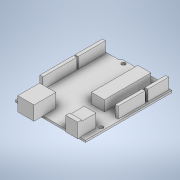
# Autodesk Inventor part: Arduino UNO
Saved by Autodesk Inventor 2020 (Build 240168000, 168)
## iProperties
Created: 2021-04-04
Part Number: Arduino UNO
Material: Типовые
Document SubType Name: Modeling
Designer: Антон
Density: 1 g/cm^3
Appearance: По умолчанию
Author: Антон
Autodesk Inventor part; units mm, degrees
ref_plane "YZ Plane" through (0, 0, 0) normal (1, 0, 0) x (0, 1, 0)
ref_plane "XZ Plane" through (0, 0, 0) normal (0, 1, 0) x (-1, 0, 0)
ref_plane "XY Plane" through (0, 0, 0) normal (0, 0, 1) x (1, 0, 0)
sketch "Эскиз1" plane through (0, 0, 0) normal (0, 1, 0) x (-1, 0, 0)
  line L0 (0, 0) -> (53.5, 0)
  line L1 (53.5, 0) -> (53.5, -66)
  line L2 (53.5, -66) -> (0, -66)
  line L3 (0, -66) -> (0, 0)
  line L4 (53.5, -66) -> (40.5, -66)
  line L5 (40.5, -66) -> (3, -66)
  line L6 (3, -66) -> (3, -67.5)
  line L7 (3, -67.5) -> (40.5, -67.5)
  line L8 (40.5, -67.5) -> (40.5, -66)
  point P0 (3, -66)
  dimension "d0" = 53.5
  dimension "d1" = 66
  dimension "d4" = 13
  dimension "d5" = 37.5
  dimension "d6" = 1.5
  constraints: 18 end point, 4 parallel, 2 horizontal, 2 perpendicular, 1 point on line
  measures "d0" distance of L1.end L2.end
  measures "d1" distance of L0.end L1.end
  measures "d4" distance of L1.end L4.end
  measures "d5" distance of L7.end L6.end
  measures "d6" distance of L5.end L6.end
extrude "Выдавливание1" add sketch "Эскиз1" along normal blind 1.5
sketch "Эскиз2" plane through (0, 1.5, 0) normal (0, 1, 0) x (1, 0, 0)
  line L0 (-40.5, 66) -> (-53.5, 66) projected
  line L1 (-53.5, 66) -> (-52, 66)
  line L2 (-52, 66) -> (-52, 65)
  line L3 (-52, 65) -> (-49.7, 65)
  line L4 (-49.7, 65) -> (-49.7, 44)
  line L5 (-49.7, 44) -> (-52, 44)
  line L6 (-52, 44) -> (-52, 65)
  line L7 (-49.7, 44) -> (-49.7, 43)
  line L8 (-49.7, 43) -> (-52, 43)
  line L9 (-52, 43) -> (-52, 17.2)
  line L10 (-52, 17.2) -> (-49.7, 17.2)
  line L11 (-49.7, 17.2) -> (-49.7, 43)
  point P0 (0, 0)
  dimension "d15" = 1.5
  dimension "d16" = 1
  dimension "d17" = 2.3
  dimension "d18" = 21
  dimension "d19" = 1
  dimension "d20" = 25.8
  constraints: 22 end point, 4 parallel, 2 horizontal, 2 perpendicular, 2 vertical, 1 point on line
  measures "d15" distance of L0.end L1.end
  measures "d16" distance of L1.end L2.end
  measures "d17" distance of L4.end L5.end
  measures "d18" distance of L3.end L4.end
  measures "d19" distance of L4.end L7.end
  measures "d20" distance of L9.end L8.end
extrude "Выдавливание2" add sketch "Эскиз2" along normal blind 8.5
sketch "Эскиз3" plane through (0, 1.5, 0) normal (0, 1, 0) x (1, 0, 0)
  line L0 (-53.5, 66) -> (-53.5, 0) projected
  line L1 (-53.5, 0) -> (-53.5, 3)
  line L2 (-53.5, 3) -> (-52.5, 3)
  line L3 (-52.5, 3) -> (-46.5, 3)
  line L4 (-46.5, 3) -> (-46.5, 9.5)
  line L5 (-46.5, 9.5) -> (-52.5, 9.5)
  line L6 (-52.5, 9.5) -> (-52.5, 3)
  point P0 (0, 0)
  dimension "d23" = 3
  dimension "d24" = 1
  dimension "d25" = 6
  dimension "d26" = 6.5
  constraints: 12 end point, 2 horizontal, 2 parallel, 1 perpendicular, 1 point on line
  measures "d23" distance of L0.end L1.end
  measures "d24" distance of L1.end L2.end
  measures "d25" distance of L5.end L4.end
  measures "d26" distance of L4.end L3.end
extrude "Выдавливание3" add sketch "Эскиз3" along normal blind 2
sketch "Эскиз4" plane through (0, 3.5, 0) normal (0, 1, 0) x (1, 0, 0)
  line L0 (-52.5, 3) -> (-52.5, 9.5) projected
  line L1 (-52.5, 6.25) -> (-46.5, 6.25)
  line L2 (-46.5, 3) -> (-46.5, 9.5) projected
  circle A0 centre (-49.5, 6.25) radius 1.5
  point P0 (0, 0)
  dimension "d29" = 3
  constraints: 3 midpoint, 2 end point, 1 centre point
  measures "d29" diameter of A0
extrude "Выдавливание4" add sketch "Эскиз4" along normal blind 0.5
sketch "Эскиз5" plane through (0, 1.5, 0) normal (0, 1, 0) x (1, 0, 0)
  line L0 (-46.5, 9.5) -> (-52.5, 9.5) projected
  line L1 (-46.5, 9.5) -> (-44.5, 9.5)
  line L2 (-44.5, 9.5) -> (-32.2, 9.5)
  line L3 (-32.2, 9.5) -> (-32.2, -7.1)
  line L4 (-32.2, -7.1) -> (-44.5, -7.1)
  line L5 (-44.5, -7.1) -> (-44.5, 9.5)
  point P0 (0, 0)
  dimension "d30" = 0.5
  dimension "d32" = 2
  dimension "d33" = 12.3
  dimension "d34" = 16.6
  constraints: 10 end point, 2 horizontal, 2 parallel, 1 perpendicular
  measures "d32" distance of L0.start L1.end
  measures "d33" distance of L3.end L4.end
  measures "d34" distance of L2.end L3.end
extrude "Выдавливание5" add sketch "Эскиз5" along normal blind 10.8
sketch "Эскиз6" plane through (0, 1.5, 0) normal (0, 1, 0) x (1, 0, 0)
  line L0 (-32.2, 0) -> (0, 0) projected
  line L1 (0, 0) -> (-4, 0)
  line L2 (-4, 0) -> (-4, 12)
  line L3 (-4, 12) -> (-13, 12)
  line L4 (-13, 12) -> (-13, -2)
  line L5 (-13, -2) -> (-4, -2)
  line L6 (-4, -2) -> (-4, 12)
  dimension "d37" = 4
  dimension "d38" = 12
  dimension "d39" = 9
  dimension "d40" = 14
  constraints: 12 end point, 2 parallel, 1 horizontal, 1 perpendicular, 1 point on line, 1 vertical
  measures "d37" distance of L0.end L1.end
  measures "d38" distance of L1.end L2.end
  measures "d39" distance of L5.end L4.end
  measures "d40" distance of L4.end L3.end
extrude "Выдавливание6" add sketch "Эскиз6" along normal blind 11
sketch "Эскиз7" plane through (0, 12.5, 0) normal (0, 1, 0) x (1, 0, 0)
  line L0 (-13, 12) -> (-13, -2) projected
  line L1 (-13, 12) -> (-4, 12)
  line L2 (-4, 12) -> (-4, 1)
  line L3 (-4, 1) -> (-13, 1)
  line L4 (-13, 1) -> (-13, 12)
  point P0 (0, 0)
  dimension "d43" = 11
  constraints: 8 end point, 2 parallel, 1 horizontal, 1 perpendicular
  measures "d43" distance of L1.end L2.end
extrude "Выдавливание7" cut sketch "Эскиз7" against normal blind 1
sketch "Эскиз8" plane through (0, 1.5, 0) normal (0, 1, 0) x (1, 0, 0)
  line L0 (0, 0) -> (0, 66) projected
  line L1 (0, 66) -> (0, 65)
  line L2 (0, 65) -> (-1.5, 65)
  line L3 (-1.5, 65) -> (-3.8, 65)
  line L4 (-3.8, 65) -> (-3.8, 49)
  line L5 (-3.8, 49) -> (-1.5, 49)
  line L6 (-1.5, 49) -> (-1.5, 65)
  line L7 (-1.5, 49) -> (-1.5, 47)
  line L8 (-1.5, 47) -> (-3.8, 47)
  line L9 (-3.8, 47) -> (-3.8, 26.5)
  line L10 (-3.8, 26.5) -> (-1.5, 26.5)
  line L11 (-1.5, 26.5) -> (-1.5, 47)
  dimension "d47" = 1
  dimension "d48" = 1.5
  dimension "d49" = 2.3
  dimension "d50" = 16
  dimension "d51" = 2
  dimension "d52" = 20.5
  constraints: 22 end point, 4 parallel, 3 horizontal, 2 perpendicular, 1 point on line, 1 vertical
  measures "d47" distance of L0.end L1.end
  measures "d48" distance of L1.end L2.end
  measures "d49" distance of L5.end L4.end
  measures "d50" distance of L4.end L3.end
  measures "d51" distance of L5.end L7.end
  measures "d52" distance of L9.end L8.end
extrude "Выдавливание8" add sketch "Эскиз8" along normal blind 8.5
sketch "Эскиз9" plane through (0, 1.5, 0) normal (0, 1, 0) x (1, 0, 0)
  line L0 (0, 0) -> (0, 66) projected
  line L1 (0, 66) -> (-21.5, 66)
  line L2 (-21.5, 66) -> (-21.5, 26)
  line L3 (-21.5, 26) -> (-11.5, 26)
  line L4 (-11.5, 26) -> (-11.5, 61.5)
  line L5 (-11.5, 61.5) -> (-21.5, 61.5)
  line L6 (-21.5, 61.5) -> (-21.5, 26)
  dimension "d55" = 21.5
  dimension "d56" = 40
  dimension "d57" = 10
  dimension "d58" = 35.5
  constraints: 12 end point, 2 horizontal, 2 parallel, 1 perpendicular, 1 vertical
  measures "d55" distance of L0.end L1.end
  measures "d56" distance of L1.end L2.end
  measures "d57" distance of L5.end L4.end
  measures "d58" distance of L4.end L3.end
extrude "Выдавливание9" add sketch "Эскиз9" along normal blind 8
sketch "Эскиз10" plane through (0, 1.5, 0) normal (0, 1, 0) x (1, 0, 0)
  line L0 (-40.5, 67.5) -> (-40.5, 66) projected
  line L1 (-40.5, 67.5) -> (-36, 67.5)
  line L2 (-3, 67.5) -> (-40.5, 67.5) projected
  line L3 (-36, 67.5) -> (-36, 65)
  line L4 (-3, 67.5) -> (-7.5, 67.5)
  line L5 (-7.5, 67.5) -> (-7.5, 65)
  line L6 (0, 0) -> (0, 14.5)
  line L7 (0, 0) -> (0, 66) projected
  line L8 (0, 14.5) -> (-2.5, 14.5)
  line L9 (-53.5, 66) -> (-53.5, 0) projected
  line L10 (-53.5, 0) -> (-53.5, 13.5)
  line L11 (-53.5, 13.5) -> (-51, 13.5)
  dimension "d67" = 4.5
  dimension "d68" = 2.5
  dimension "d69" = 4.5
  dimension "d70" = 2.5
  dimension "d71" = 14.5
  dimension "d72" = 2.5
  dimension "d73" = 13.5
  dimension "d74" = 2.5
  constraints: 16 end point, 4 point on line, 3 perpendicular, 1 vertical
  measures "d67" distance of L0.start L1.end
  measures "d68" distance of L1.end L3.end
  measures "d69" distance of L2.start L4.end
  measures "d70" distance of L4.end L5.end
  measures "d71" distance of L6.start L6.end
  measures "d72" distance of L6.end L8.end
  measures "d73" distance of L9.end L10.end
  measures "d74" distance of L10.end L11.end
hole "Отверстие1" at (-51, 1.5, -13.5) at (-2.5, 1.5, -14.5) at (-7.5, 1.5, -65) at (-36, 1.5, -65) direction (0, -1, 0) diameter 3 end through all
chamfer "Фаска3" distance 1.5 angle 45 2 edges at (-40.5, 0.75, -67.5) (-3, 0.75, -67.5)
chamfer "Фаска4" distance 1 angle 45 1 edges at (-53.5, 0.75, -66)
